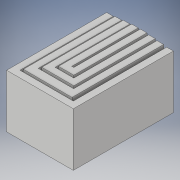
# Autodesk Inventor part: rectangle lift idea
Saved by Autodesk Inventor 2017 (Build 210142000, 142)
## iProperties
Created: 2017-08-30
Part Number: rectangle lift idea
Material: Generic
Document SubType Name: Modeling
Designer: User
Density: 1 g/cm^3
Appearance: Default
Author: User
Autodesk Inventor part; units mm, degrees
ref_plane "YZ Plane" through (0, 0, 0) normal (1, 0, 0) x (0, 1, 0)
ref_plane "XZ Plane" through (0, 0, 0) normal (0, 1, 0) x (-1, 0, 0)
ref_plane "XY Plane" through (0, 0, 0) normal (0, 0, 1) x (1, 0, 0)
sketch "Sketch1" plane through (0, 0, 0) normal (0, 1, 0) x (-1, 0, 0)
  line L0 (0, 0) -> (508, 0)
  line L1 (508, 0) -> (508, -50.8)
  line L2 (508, -50.8) -> (0, -50.8)
  line L3 (0, -50.8) -> (0, 0)
  line L4 (0, 0) -> (50.8, 0)
  line L5 (50.8, 0) -> (50.8, -762)
  line L6 (50.8, -762) -> (0, -762)
  line L7 (0, -762) -> (0, 0)
  line L8 (508, 0) -> (457.2, 0)
  line L9 (457.2, 0) -> (457.2, -762)
  line L10 (457.2, -762) -> (508, -762)
  line L11 (508, -762) -> (508, 0)
  line L12 (50.8, -762) -> (457.2, -762)
  line L13 (324.0208, -50.8) -> (324.0208, -63.5)
  line L14 (457.2, -242.977) -> (444.5, -242.977)
  line L15 (50.8, -225.2641) -> (63.5, -225.2641)
  dimension "d0" = 508
  dimension "d1" = 50.8
  dimension "d2" = 50.8
  dimension "d3" = 762
  dimension "d4" = 50.8
  dimension "d5" = 762
  dimension "d6" = 12.7
  dimension "d7" = 12.7
  dimension "d8" = 12.7
  constraints: 32 end point, 6 parallel, 6 perpendicular, 3 horizontal, 3 point on line
  measures "d0" distance of L1.end L2.end
  measures "d1" distance of L0.end L1.end
  measures "d2" distance of L5.end L6.end
  measures "d3" distance of L4.end L5.end
  measures "d4" distance of L10.end L9.end
  measures "d5" distance of L9.end L8.end
  measures "d6" distance of L13.start L13.end
  measures "d7" distance of L14.start L14.end
  measures "d8" distance of L15.start L15.end
sketch "Sketch2" plane through (0, 0, 0) normal (0, 1, 0) x (-1, 0, 0)
  line L0 (444.4154, -126.9138) -> (394.1877, -126.9138)
  line L1 (73.5741, -107.6392) -> (73.5741, -94.9392)
  line L2 (50.8, -762) -> (457.2, -762) projected
  line L3 (324.0208, -50.8) -> (324.0208, -63.5) projected
  line L4 (444.4154, -126.9138) -> (73.5741, -126.9138)
  line L5 (73.5741, -126.9138) -> (73.5741, -63.5)
  line L6 (73.5741, -63.5) -> (444.4154, -63.5)
  line L7 (444.4154, -63.5) -> (444.4154, -126.9138)
  line L8 (73.5741, -762) -> (124.3741, -762)
  line L9 (124.3741, -762) -> (124.3741, -126.9138)
  line L10 (124.3741, -63.5) -> (73.5741, -63.5)
  line L11 (73.5741, -63.5) -> (73.5741, -762)
  line L12 (444.4154, -63.5) -> (393.6154, -63.5)
  line L13 (393.6154, -126.9138) -> (393.6154, -762)
  line L14 (393.6154, -762) -> (444.4154, -762)
  line L15 (444.4154, -762) -> (444.4154, -63.5)
  point P0 (0, 0)
  dimension "d31" = 50.8
  dimension "d32" = 50.8
  constraints: 28 end point, 6 parallel, 5 point on line, 4 horizontal, 3 perpendicular, 1 coincident
  measures "d31" distance of L10.end L10.start
  measures "d32" distance of L14.end L13.end
sketch "Sketch3" plane through (0, 0, 0) normal (0, 1, 0) x (-1, 0, 0)
  line L0 (266.2128, -127.9629) -> (266.2128, -140.6629)
  line L1 (393.6154, -126.9138) -> (393.6154, -762) projected
  line L2 (124.3741, -762) -> (124.3741, -126.9138) projected
  line L3 (124.3741, -238.3365) -> (137.0741, -238.3365)
  line L4 (393.6154, -256.759) -> (380.9154, -256.759)
  line L5 (137.0741, -762) -> (187.8741, -762)
  line L6 (187.8741, -762) -> (187.8741, -140.6629)
  line L7 (187.8741, -140.6629) -> (137.0741, -140.6629)
  line L8 (137.0741, -140.6629) -> (137.0741, -762)
  line L9 (187.8741, -140.6629) -> (380.9154, -140.6629)
  line L10 (380.9154, -140.6629) -> (380.9154, -191.4629)
  line L11 (380.9154, -191.4629) -> (187.8741, -191.4629)
  line L12 (187.8741, -191.4629) -> (187.8741, -140.6629)
  line L13 (380.9154, -191.4629) -> (330.1154, -191.4629)
  line L14 (330.1154, -191.4629) -> (330.1154, -762)
  line L15 (330.1154, -762) -> (380.9154, -762)
  line L16 (380.9154, -762) -> (380.9154, -191.4629)
  line L17 (266.2128, -191.4629) -> (266.2128, -204.1629)
  line L18 (330.1154, -311.7256) -> (317.4154, -311.7256)
  line L19 (187.8741, -311.7256) -> (200.5741, -311.7256)
  line L20 (317.4154, -204.1629) -> (200.5741, -204.1629)
  line L21 (200.5741, -204.1629) -> (200.5741, -254.9629)
  line L22 (200.5741, -254.9629) -> (317.4154, -254.9629)
  line L23 (317.4154, -254.9629) -> (317.4154, -204.1629)
  line L24 (317.4154, -254.9629) -> (266.6154, -254.9629)
  line L25 (266.6154, -254.9629) -> (266.6154, -762)
  line L26 (266.6154, -762) -> (317.4154, -762)
  line L27 (317.4154, -762) -> (317.4154, -254.9629)
  line L28 (200.5741, -254.9629) -> (251.3741, -254.9629)
  line L29 (251.3741, -254.9629) -> (251.3741, -762)
  line L30 (251.3741, -762) -> (200.5741, -762)
  line L31 (200.5741, -762) -> (200.5741, -254.9629)
  point P0 (0, 0)
  dimension "d33" = 12.7
  dimension "d34" = 12.7
  dimension "d35" = 12.7
  dimension "d36" = 50.8
  dimension "d37" = 50.8
  dimension "d38" = 50.8
  dimension "d39" = 12.7
  dimension "d40" = 12.7
  dimension "d41" = 12.7
  dimension "d42" = 50.8
  dimension "d43" = 50.8
  dimension "d44" = 50.8
  constraints: 60 end point, 12 parallel, 9 perpendicular, 7 horizontal, 6 point on line, 2 vertical
  measures "d33" distance of L0.start L0.end
  measures "d34" distance of L3.start L3.end
  measures "d35" distance of L4.start L4.end
  measures "d36" distance of L7.end L6.end
  measures "d37" distance of L9.end L10.end
  measures "d38" distance of L15.end L14.end
  measures "d39" distance of L17.start L17.end
  measures "d40" distance of L18.start L18.end
  measures "d41" distance of L19.start L19.end
  measures "d42" distance of L21.end L20.end
  measures "d43" distance of L26.end L25.end
  measures "d44" distance of L29.end L30.end
extrude "Extrusion1" add sketch "Sketch1" along normal blind 406.4 contours L0 L5 L2 L3 | L0 L9 L2 L5 | L2 L5 L6 L7 | L0 L1 L2 L9 | L2 L11 L10 L9
extrude "Extrusion2" add sketch "Sketch2" along normal blind 412.75 contours L15 L2 L13 L4 L0 | L0 L4 L5 L1 L6 L7 | L9 L2 L11 L4
extrude "Extrusion3" add sketch "Sketch3" along normal blind 419.1 contours L8 L7 L6 L5 | L6 L9 L10 L11 | L11 L16 L15 L14
extrude "Extrusion4" add sketch "Sketch3" along normal blind 425.45 contours L31 L22 L29 L30 | L21 L20 L23 L22 | L22 L27 L26 L25
body "Solid1"
